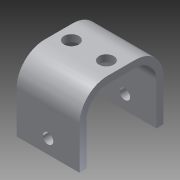
# Autodesk Inventor part: pulley mount
Saved by Autodesk Inventor 2013 (Build 170138000, 138)
## iProperties
Created: 2013-01-27
Part Number: pulley mount
Material: Aluminum 6061
Document SubType Name: Sheet Metal
Designer: Arpan
Density: 1 g/cm^3
Sheet Metal Rule: Default
Author: Arpan
Autodesk Inventor part; units mm, degrees
ref_plane "YZ Plane" through (0, 0, 0) normal (1, 0, 0) x (0, 1, 0)
ref_plane "XZ Plane" through (0, 0, 0) normal (0, 1, 0) x (-1, 0, 0)
ref_plane "XY Plane" through (0, 0, 0) normal (0, 0, 1) x (1, 0, 0)
sketch "Sketch1" plane through (0, 0, 0) normal (0, 0, 1) x (1, 0, 0)
  line L0 (0, 0) -> (-28.575, 0)
  line L1 (-28.575, 0) -> (-28.575, 19.05)
  line L2 (-28.575, 19.05) -> (0, 19.05)
  line L3 (0, 19.05) -> (0, 0)
  line L4 (-14.2875, 0) -> (-14.2875, 6.35)
  circle A0 centre (-14.2875, 6.35) radius 2.3812
  dimension "d0" = 28.575
  dimension "d1" = 19.05
  dimension "d2" = 6.35
  dimension "d3" = 4.7625
  measures "d0" distance of L0.start L0.end
  measures "d1" distance of L0.end L1.end
  measures "d2" distance of L4.start L4.end
  measures "d3" diameter of A0
extrude "Plate1" add sketch "Sketch1" along normal blind 3.175
sketch "Sketch5" plane through (0, 28.575, -9.525) normal (0, 1, 0) x (-1, 0, 0)
  line L0 (28.575, 0) -> (0, 0)
  line L1 (0, 0) -> (0, -12.7)
  line L2 (0, -12.7) -> (28.575, -12.7)
  line L3 (28.575, -12.7) -> (28.575, 0)
  constraints: 6 end point, 1 horizontal, 1 perpendicular, 1 vertical
edge flange "Flange3" height 25.4 angle 90 thickness 3.175 bend radius 9.525 thickness toward (0, 1, 0) relief straight relief width 3.175 relief depth 1.5875 edges at (-14.2875, 19.05, 0) wall of the first edge with corners at (-28.575, 28.575, -9.525) (0, 28.575, -9.525) (0, 28.575, -22.225) (-28.575, 28.575, -22.225)
bend "Bend3"
corner "Corner3"
sketch "Sketch6" plane through (0, 19.05, -31.75) normal (0, 0, -1) x (-1, 0, 0)
  line L0 (28.575, 0) -> (0, 0)
  line L1 (0, 0) -> (0, -19.05)
  line L2 (0, -19.05) -> (28.575, -19.05)
  line L3 (28.575, -19.05) -> (28.575, 0)
  constraints: 6 end point, 1 horizontal, 1 perpendicular, 1 vertical
edge flange "Flange4" height 31.75 angle 90 thickness 3.175 bend radius 9.525 thickness toward (0, 0, -1) relief straight relief width 3.175 relief depth 1.5875 edges at (-14.2875, 28.575, -22.225) wall of the first edge with corners at (-28.575, 19.05, -31.75) (0, 19.05, -31.75) (0, 0, -31.75) (-28.575, 0, -31.75)
bend "Bend4"
corner "Corner4"
sketch "Sketch7" plane through (0, 0, -34.925) normal (0, 0, -1) x (-1, 0, 0)
  circle A0 centre (14.2875, 6.35) radius 2.3812 projected
  circle A1 centre (14.2875, 6.35) radius 2.3812 projected
extrude "Cut2" cut sketch "Sketch7" against normal blind 3.175
sketch "Sketch8" plane through (-28.575, 31.75, -9.525) normal (0, 1, 0) x (1, 0, 0)
  line L0 (28.575, 12.7) -> (28.575, 0) projected
  line L1 (0, 0) -> (0, 12.7) projected
  line L2 (0, 5.8436) -> (6.35, 5.8436)
  circle A0 centre (6.35, 5.8436) radius 3.3782
  line L3 (28.575, 5.8436) -> (22.225, 5.8436)
  circle A1 centre (22.225, 5.8436) radius 3.3782
  point P0 (28.575, -9.525)
  dimension "d51" = 6.35
  dimension "d52" = 6.7564
  dimension "d53" = 6.35
  dimension "d54" = 6.7564
  constraints: 4 end point, 2 centre point, 2 coincident, 2 point on line, 1 collinear, 1 perpendicular
  measures "d51" distance of L2.start L2.end
  measures "d52" diameter of A0
  measures "d53" distance of L3.start L3.end
  measures "d54" diameter of A1
extrude "Cut3" cut sketch "Sketch8" against normal blind 3.175
sketch "Sketch9" plane through (-28.575, 31.75, -9.525) normal (0, 1, 0) x (1, 0, 0)
  circle A0 centre (6.35, 5.8436) radius 3.3782 projected
  circle A1 centre (22.225, 5.8436) radius 3.3782 projected
  line L0 (0, 0) -> (28.575, 0) projected
  line L1 (28.575, 12.7) -> (28.575, 0) projected
  line L2 (0, 12.7) -> (28.575, 12.7) projected
  line L3 (0, 0) -> (0, 12.7) projected
  point P0 (28.575, -9.525)
equation "\"d49\" = Thickness"
equation "\"d55\" = Thickness"
equation "\"d29\" = BendReliefWidth"
equation "\"d30\" = BendReliefDepth"
equation "\"d31\" = MinimumRemnant"
equation "\"d32\" = BendRadius"
equation "\"d36\" = CornerReliefSize"
equation "\"d37\" = GapSize"
equation "\"d38\" = JacobiRadiusSize"
equation "\"d39\" = BendReliefWidth"
equation "\"d40\" = BendReliefDepth"
equation "\"d41\" = MinimumRemnant"
equation "\"d42\" = BendRadius"
equation "\"d46\" = CornerReliefSize"
equation "\"d47\" = GapSize"
equation "\"d48\" = JacobiRadiusSize"
equation "\"BendRadius\" = Thickness"
equation "\"BendReliefWidth\" = Thickness"
equation "\"BendReliefDepth\" = 0.5 * Thickness"
equation "\"CornerReliefSize\" = 4 * Thickness"
equation "\"MinimumRemnant\" = 2 * Thickness"
equation "\"TransitionRadius\" = BendRadius"
equation "\"JacobiRadiusSize\" = BendRadius"
equation "\"GapSize\" = Thickness"
equation "\"d4\" = BendRadius"
equation "\"Thickness\" = 3.175"
body "Solid1"
